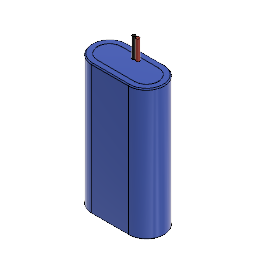
354 4400mah battery (Autodesk Fusion 360 design; units mm, degrees)
Autodesk Fusion 360 part; units mm, degrees
sketch "Sketch1" plane through (0, 0, 0) normal (0, 0, 1) x (1, 0, 0)
  line L0 (-9.3, -9) -> (9.3, -9)
  arc A0 (9.3, -9) -> (9.3, 9) centre (9.3, 0) ccw
  line L1 (9.3, 9) -> (-9.3, 9)
  arc A1 (-9.3, 9) -> (-9.3, -9) centre (-9.3, 0) ccw
  line L2 (-9.3, 0) -> (9.3, 0) construction
  line L3 (-18, -17.3925) -> (18, -17.3925) construction
  line L4 (0, -17.3925) -> (0, 0)
  arc A2 (9.3, -6) -> (9.3, 6) centre (9.3, 0) ccw
  line L5 (9.3, 6) -> (-9.3, 6)
  arc A3 (-9.3, 6) -> (-9.3, -6) centre (-9.3, 0) ccw
  line L6 (-9.3, -6) -> (9.3, -6)
  dimension "d1" = 18
  dimension "d2" = 18.6
  dimension "d3" = 36
  dimension "d6" = 3
  measures "d1" diameter of A0
extrude "Extrude1" add sketch "Sketch1" along normal blind 66 makes body 1
extrude "Extrude2" add sketch "Sketch1" along normal up to surface (66 mm away) separate body contours A2 L5 A3 L6 makes body 2
fillet "Fillet1" radius 0.5 8 edges at (18.3, 0, 66) (0, 9, 66) (-18.3, 0, 66) (0, -9, 66) (18.3, 0, 0) (0, 9, 0) (-18.3, 0, 0) (0, -9, 0) on bodies 1
sketch "Sketch2" plane through (0, 0, 66) normal (0, 0, 1) x (-1, 0, 0)
  arc A0 (9.3, -6) -> (9.3, 6) centre (9.3, 0) ccw
  line L0 (9.3, 6) -> (-9.3, 6)
  arc A1 (-9.3, 6) -> (-9.3, -6) centre (-9.3, 0) ccw
  line L1 (-9.3, -6) -> (9.3, -6)
  circle A2 centre (1, -4) radius 0.85
  circle A3 centre (-1, -4) radius 0.85
  line L2 (-1, -4) -> (1, -4) construction
  line L3 (0, -4) -> (0, 0)
  dimension "d10" = 1.7
  dimension "d11" = 1.7
  dimension "d12" = 2
  measures "d10" diameter of A2
  measures "d11" diameter of A3
extrude "Extrude3" add sketch "Sketch2" along normal blind 10 separate body contours A2 | A3 makes body 3 at (-1.8489, 4.0424, 72.6667) makes body 4 at (0.1511, 4.0424, 72.6667)
